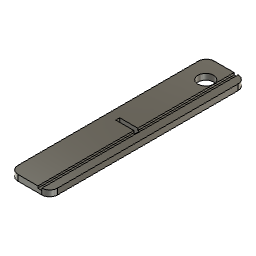
filament-gauge (Autodesk Fusion 360 design; units mm, degrees)
Autodesk Fusion 360 part; units mm, degrees
sketch "Sketch1" plane through (0, 0, 0) normal (0, 0, 1) x (1, 0, 0)
  line L0 (0, 0) -> (20.2, 0)
  line L1 (20.2, 0) -> (20.2, 100.2)
  line L2 (20.2, 100.2) -> (0, 100.2)
  line L3 (0, 100.2) -> (0, 0)
  circle A0 centre (10.1, 89.7864) radius 4
  line L4 (15, 51) -> (5, 51)
  line L5 (5, 51) -> (5, 49)
  line L6 (5, 49) -> (15, 49)
  line L7 (15, 49) -> (15, 51)
  line L8 (15, 51) -> (5, 49) construction
  line L9 (5, 51) -> (15, 49) construction
  line L10 (10.1, 100.2) -> (10.1, 0) construction
  point P0 (10, 50)
  dimension "d1" = 20.2
  dimension "d2" = 100.2
  dimension "d8" = 8
  dimension "d9" = 10
  dimension "d10" = 2
  constraint horizontal L0
  constraint vertical L1
  constraint horizontal L2
  constraint vertical L3
  constraint coincident L0.start L3.end
  constraint horizontal L4
  constraint perpendicular L4 L5
  constraint parallel L4 L6
  constraint parallel L5 L7
  constraint coincident L8 P0
  constraint coincident L9 P0
  constraint midpoint L2 L10.start
  constraint midpoint L0 L10.end
  constraint coincident A0.centre L10
  measures "d1" distance of L0.start L0.end
  measures "d2" distance of L0.start L2.end
  measures "d8" diameter of A0
  measures "d9" distance of L5.end L6.end
  measures "d10" distance of L4.end L5.end
extrude "Extrude1" add sketch "Sketch1" along normal blind 3
fillet "Fillet1" radius 4 4 edges at (20.2, 0, 1.5) (20.2, 100.2, 1.5) (0, 100.2, 1.5) (0, 0, 1.5)
sketch "Sketch2" plane through (0, 0, 3) normal (0, 0, 1) x (-1, 0, 0)
  arc A0 (0, -4) -> (-4, 0) centre (-4, -4) ccw
  line L0 (-4, 0) -> (-16.2, 0)
  arc A1 (-16.2, 0) -> (-20.2, -4) centre (-16.2, -4) ccw
  line L1 (-20.2, -4) -> (-20.2, -96.2)
  arc A2 (-20.2, -96.2) -> (-16.2, -100.2) centre (-16.2, -96.2) ccw
  line L2 (-16.2, -100.2) -> (-4, -100.2)
  arc A3 (-4, -100.2) -> (0, -96.2) centre (-4, -96.2) ccw
  line L3 (0, -96.2) -> (0, -4)
  line L4 (-15, -51) -> (-15, -49)
  line L5 (-15, -49) -> (-5, -49)
  line L6 (-5, -49) -> (-5, -51)
  line L7 (-5, -51) -> (-15, -51)
  circle A4 centre (-10.1, -89.7864) radius 4
  line L8 (-16.2, 0) -> (-14.2, 0)
  line L9 (-14.2, 0) -> (-14.2, -100.2)
  line L10 (-14.2, -100.2) -> (-16.2, -100.2)
  line L11 (-16.2, -100.2) -> (-16.2, 0)
  dimension "d11" = 2
  constraint horizontal L8
  constraint vertical L9
  constraint horizontal L10
  constraint vertical L11
  constraint coincident L0.end A1.start
  measures "d11" distance of L0.end L8.end
extrude "Extrude2" cut sketch "Sketch2" against normal blind 1 contours L0 L2 L4 L5 L7 L8 L9 L10 L11
